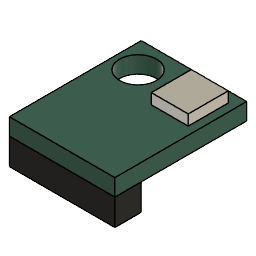
GREENHOUSE NEW VERSION (Autodesk Fusion 360 archive; units mm, degrees)
design "BMP180"
Autodesk Fusion 360 part; units mm, degrees
(part 1 of 25)
sketch "Sketch1" plane through (0, 0, 0) normal (0, 0, 1) x (1, 0, 0)
  line L0 (0, 0) -> (10, 0)
  line L1 (10, 0) -> (10, 12.5)
  line L2 (10, 12.5) -> (0, 12.5)
  line L3 (0, 12.5) -> (0, 0)
  circle A0 centre (2.25, 9.95) radius 1.75
  line L4 (5.75, 11.5) -> (9.25, 11.5)
  line L5 (9.25, 11.5) -> (9.25, 7.7)
  line L6 (9.25, 7.7) -> (5.75, 7.7)
  line L7 (5.75, 7.7) -> (5.75, 11.5)
  line L8 (10, 2.5) -> (0, 2.5)
  dimension "d1" = 10
  dimension "d2" = 12.5
  dimension "d3" = 3.5
  dimension "d4" = 2.55
  dimension "d5" = 2.25
  dimension "d6" = 3.5
  dimension "d7" = 3.8
  dimension "d8" = 0.75
  dimension "d9" = 1
  dimension "d10" = 2.5
  constraint horizontal L0
  constraint vertical L1
  constraint horizontal L2
  constraint vertical L3
  constraint coincident L0.start L3.end
  constraint horizontal L4
  constraint vertical L5
  constraint horizontal L6
  constraint vertical L7
  constraint coincident L1 L8.start
  constraint coincident L3 L8.end
  constraint perpendicular L3 L8
  measures "d1" distance of L0.start L0.end
  measures "d2" distance of L0.start L2.end
  measures "d3" diameter of A0
  measures "d4" distance of L2 A0.centre
  measures "d5" distance of L3 A0.centre
  measures "d6" distance of L4.start L4.end
  measures "d7" distance of L4.start L6.end
  measures "d8" distance of L1 L5
  measures "d9" distance of L2 L4
  measures "d10" distance of L0 L8
extrude "Extrude1" add sketch "Sketch1" along normal blind 1.6 contours L0 L1 L3 L8 | L1 L2 L3 L8 | L4 L5 L6 L7 makes body 1
extrude "Extrude2" add sketch "Sketch1" along normal blind 1 from surface at 1.6 separate body contours L4 L5 L6 L7 makes body 2
extrude "Extrude3" add sketch "Sketch1" against normal blind 2.5 separate body contours L0 L1 L3 L8 makes body 3
equation "d4 = d3 / 2 + 0.8 mm"
equation "d5 = d3 / 2 + 0.5 mm"

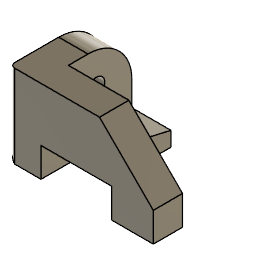
design "MOUNT REAl"
part number: 2026-05-05-22-33-46-720
Autodesk Fusion 360 part; units mm, degrees
sketch "Sketch1" plane through (0, 0, 0) normal (0, 0, 1) x (1, 0, 0)
  line L0 (0, 0) -> (14.68, 0)
  line L1 (14.68, 0) -> (14.68, 3)
  line L2 (14.68, 3) -> (11.68, 3)
  line L3 (11.68, 3) -> (3, 3)
  line L4 (3, 3) -> (3, 9.502)
  line L5 (0, 0) -> (0, 9.502)
  line L6 (0, 9.502) -> (3, 9.502)
  dimension "d4" = 3
  dimension "d5" = 3
  dimension "d6" = 8.68
  dimension "d7" = 6.502
  dimension "d88" = 3
  constraint coincident L0.start L5.start
  constraint horizontal L0
  constraint perpendicular L0 L1
  constraint perpendicular L1 L2
  constraint parallel L2 L3
  constraint perpendicular L3 L4
  constraint perpendicular L0 L5
  constraint perpendicular L4 L6
  measures "d4" distance of L0.end L1.end
  measures "d5" distance of L1.end L2.end
  measures "d6" distance of L2.end L3.end
  measures "d7" distance of L3.end L4.end
  measures "d88" distance of L4.end L5.end
extrude "Extrude18" add sketch "Sketch1" along normal blind 8.5 makes body 1
sketch "Sketch18" plane through (0, 0, 0) normal (0, -1, 0) x (1, 0, 0)
  line L0 (0, 0) -> (14.68, 0)
  line L1 (14.68, 0) -> (14.68, 8.5)
  line L2 (14.68, 8.5) -> (0, 8.5)
  line L3 (0, 8.5) -> (0, 0)
  line L4 (3.2, 0) -> (10.41, 0)
  line L5 (10.41, 0) -> (10.41, 3)
  line L6 (10.41, 3) -> (3.2, 3)
  line L7 (3.2, 3) -> (3.2, 0)
  dimension "d93" = 7.21
  dimension "d94" = 3
  dimension "d95" = 10.41
  constraint perpendicular L4 L5
  constraint perpendicular L5 L6
  constraint perpendicular L4 L7
  constraint coincident L0 L4.start
  constraint coincident L0 L4.end
  measures "d93" distance of L5.end L6.end
  measures "d94" distance of L4.end L5.end
  measures "d95" distance of L3 L5
extrude "Extrude19" cut sketch "Sketch18" against normal blind 3 contours L0 L4 L5 L6 L7 bodies 1
sketch "Sketch19" plane through (0, 0, 0) normal (0, 0, 1) x (1, 0, 0)
  line L0 (1.73, 2) -> (1.73, 8.5)
  line L1 (1.73, 8.5) -> (7.43, 8.5)
  line L2 (7.43, 8.5) -> (7.43, 2)
  line L3 (7.43, 2) -> (1.73, 2)
  dimension "d99" = 5.7
  constraint perpendicular L0 L1
  constraint perpendicular L1 L2
  measures "d99" distance of L0.end L1.end
sketch "Sketch23" plane through (0, 0, 0) normal (-1, 0, 0) x (0, -1, 0)
  line L0 (-9.502, 0) -> (0, 0)
  line L1 (0, 0) -> (0, 8.5)
  line L2 (0, 8.5) -> (-9.502, 8.5)
  line L3 (-9.502, 8.5) -> (-9.502, 0)
  circle A0 centre (-5.852, 5.15) radius 0.8695
  dimension "d107" = 1.739
  dimension "d108" = 3.35
  dimension "d109" = 3.65
  measures "d107" diameter of A0
  measures "d108" distance of L2 A0.centre
  measures "d109" distance of L3 A0.centre
extrude "Extrude23" cut sketch "Sketch23" against normal blind 6.5 contours A0 bodies 1
fillet "Fillet3" radius 4.5 1 edges at (1.5, 9.502, 8.5) on bodies 1
chamfer "Chamfer3" distance 0.5 angle 45 1 edges at (0, 4.751, 0) on bodies 1
fillet "Fillet4" radius 0.5 1 edges at (0, 0, 4.5) on bodies 1
chamfer "Chamfer4" distance 5.5 angle 45 1 edges at (14.68, 1.5, 8.5) on bodies 1
sketch "Sketch24" plane through (0, 0, 0) normal (0, 0, 1) x (1, 0, 0)
  line L0 (3, 3) -> (7, 3)
  line L1 (7, 3) -> (7, 9.5)
  line L2 (7, 9.5) -> (3, 9.5)
  line L3 (3, 9.5) -> (3, 3)
  dimension "d118" = 4
  dimension "d119" = 6.5
  dimension "d120" = 3
  dimension "d121" = 3
  constraint horizontal L0
  constraint perpendicular L0 L1
  constraint perpendicular L1 L2
  constraint perpendicular L0 L3
  measures "d118" distance of L0.start L0.end
  measures "d119" distance of L0 L2
  measures "d120" distance of origin L3
  measures "d121" distance of origin L0
extrude "Extrude24" add sketch "Sketch24" along normal blind 3 separate body makes body 2
sketch "Sketch25" plane through (7, 0, 0) normal (1, 0, 0) x (0, 1, 0)
  line L0 (3, 0) -> (9.5, 0)
  line L1 (9.5, 0) -> (9.5, 3)
  line L2 (9.5, 3) -> (3, 3)
  line L3 (3, 3) -> (3, 0)
  line L4 (3, 3) -> (9.5, 1.5)
  line L5 (9.5, 1.5) -> (3, 1.5)
  line L6 (3, 3) -> (3, 1.5)
  constraint coincident L2.end L3.start
  constraint midpoint L1 L4.end
  constraint midpoint L3 L5.end
extrude "Extrude25" cut sketch "Sketch25" against normal blind 2 contours L1 L2 L4 bodies 2
extrude "Extrude26" cut sketch "Sketch25" against normal blind 4 contours L1 L2 L4 bodies 2

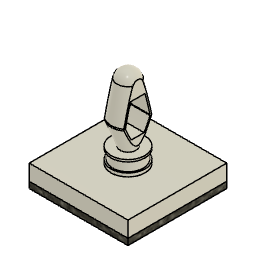
design "PCB Support Pin"
Autodesk Fusion 360 part; units mm, degrees
sketch "Sketch1" plane through (0, 0, 0) normal (0, 0, 1) x (1, 0, 0)
  line L0 (6.35, 6.35) -> (-6.35, 6.35)
  line L1 (-6.35, 6.35) -> (-6.35, -6.35)
  line L2 (-6.35, -6.35) -> (6.35, -6.35)
  line L3 (6.35, -6.35) -> (6.35, 6.35)
  line L4 (6.35, 6.35) -> (-6.35, -6.35) construction
  line L5 (-6.35, 6.35) -> (6.35, -6.35) construction
  dimension "d1" = 12.7
  dimension "d2" = 12.7
  constraint horizontal L0
  constraint perpendicular L0 L1
  constraint parallel L0 L2
  constraint parallel L1 L3
  constraint coincident L4 origin
  constraint coincident L5 origin
  measures "d1" distance of L1.end L2.end
  measures "d2" distance of L0.end L1.end
extrude "Extrude1" add sketch "Sketch1" along normal blind 2.032 makes body 1
extrude "Extrude2" add 1 faces at (-2.1167, -2.1167, 0) along direction (0, 0, -1) blind 0.8 separate body on bodies 1 makes body 2
sketch "Sketch2" plane through (0, 0, 0) normal (0, 1, 0) x (1, 0, 0)
  line L0 (-6.35, -2.032) -> (6.35, -2.032)
  line L1 (0, -2.032) -> (0, -12.6938)
  line L2 (0, -3.9625) -> (2.1828, -3.9625)
  line L3 (2.1828, -3.9625) -> (2.1828, -3.6971)
  line L4 (2.1828, -3.6971) -> (1.9857, -3.6971)
  line L5 (1.9857, -3.6971) -> (1.9857, -2.4654)
  line L6 (1.9857, -2.4654) -> (2.1828, -2.4654)
  line L7 (2.1828, -2.4654) -> (2.1828, -2.032)
  line L8 (6.35, 0.8) -> (-6.35, 0.8) construction
  line L9 (1.0176, -3.9625) -> (2.1587, -7.0975)
  line L10 (2.1763, -7.3064) -> (1.4028, -11.5248)
  arc A0 (0, -12.6938) -> (1.4028, -11.5248) centre (0, -11.2676) ccw
  arc A1 (2.1763, -7.3064) -> (2.1587, -7.0975) centre (1.7828, -7.2343) ccw
  line L11 (0, -12.6938) -> (1.1885, -12.6938) construction
  line L12 (1.1885, -12.6938) -> (1.4028, -11.5248) construction
  line L13 (2.1828, -3.9625) -> (2.1828, -7.2343) construction
  line L14 (1.6, -3.9625) -> (1.6, -5.5625) construction
  line L15 (1.6, -5.5625) -> (0, -5.5625) construction
  arc A2 (1.9795, -7.2704) -> (1.9708, -7.1659) centre (1.7828, -7.2343) ccw
  line L16 (0.8297, -4.0309) -> (0.8048, -3.9625)
  dimension "d7" = 4.7625
  dimension "d8" = 4.3656
  dimension "d10" = 0.4
  dimension "d11" = 8.7313
  dimension "d12" = 3.2
  dimension "d13" = 1.6
  dimension "d15" = 70
  constraint midpoint L0 L1.start
  constraint perpendicular L0 L1
  constraint perpendicular L1 L2
  constraint perpendicular L2 L3
  constraint perpendicular L3 L4
  constraint perpendicular L4 L5
  constraint perpendicular L5 L6
  constraint coincident L0 L7.end
  constraint perpendicular L0 L7
  constraint collinear L3 L7
  constraint coincident L2.start L1
  constraint coincident L1.end A0.start
  constraint tangent L10 A0
  constraint tangent L9 A1
  constraint tangent L10 A1
  constraint perpendicular L1 L11
  constraint tangent A0 L12
  constraint tangent A0 L11
  constraint coincident A1 L13.end
  constraint tangent A1 L13
  constraint perpendicular L2 L13
  constraint coincident L2 L9.start
  constraint coincident L2 L14.start
  constraint coincident L9 L14.end
  constraint perpendicular L2 L14
  constraint coincident L1 L15.end
  constraint perpendicular L1 L15
  constraint coincident L2 L16.end
  constraint concentric A1 A2
  measures "d7" distance of L2 L8
  measures "d10" radius of A1
  measures "d11" distance of L2 L1.end
  measures "d13" distance of L14.start L14.end
  measures "d15" angle of L2 L9
revolve "Revolve1" add sketch "Sketch2" angle 360 about axis through (0, 0, 2.032) along (0, 0, 1) bodies 1
sketch "Sketch3" plane through (0, 0, 0) normal (0, 1, 0) x (1, 0, 0)
  line L0 (-2.1828, -3.9625) -> (2.1828, -3.9625)
  arc A0 (-1.4028, -11.5248) -> (0, -12.6938) centre (0, -11.2676) ccw
  arc A1 (0, -12.6938) -> (1.4028, -11.5248) centre (0, -11.2676) ccw
  line L1 (1.25, -3.9625) -> (1.25, -12.6938)
  line L2 (1.25, -12.6938) -> (-1.25, -12.6938)
  line L3 (-1.25, -12.6938) -> (-1.25, -3.9625)
  line L4 (2.1828, -3.9625) -> (2.1828, -12.6938)
  line L5 (2.1828, -12.6938) -> (1.25, -12.6938)
  line L6 (-1.25, -12.6938) -> (-2.1828, -12.6938)
  line L7 (-2.1828, -12.6938) -> (-2.1828, -3.9625)
  dimension "d16" = 2.5
  constraint coincident L0 L1.start
  constraint perpendicular L0 L1
  constraint perpendicular L1 L2
  constraint coincident L0 L3.end
  constraint perpendicular L0 L3
  constraint midpoint A0.end L2
  constraint coincident L0.end L4.start
  constraint perpendicular L0 L4
  constraint perpendicular L1 L5
  constraint perpendicular L3 L6
  constraint coincident L0.start L7.end
  constraint perpendicular L0 L7
  measures "d16" distance of L1.end L2.end
extrude "Extrude3" cut sketch "Sketch3" along normal through all and the other way through all contours L0 L3 L6 L7 | L0 L1 L4 L5 bodies 1
sketch "Sketch4" plane through (1.25, 0, 0) normal (1, 0, 0) x (0, 1, 0)
  arc A0 (0.6367, 11.5248) -> (-0.6367, 11.5248) centre (0, 11.2676) ccw
  spline S0 degree 2 poles (-1.7815, 7.3064) (-1.0854, 10.4141) (-0.6367, 11.5248) knots 0 0 0 0.437351 0.437351 0.437351 weights 1 1.055449 1
  spline S1 degree 3 poles (-1.76, 7.0975) (-1.7782, 7.1383) (-1.7895, 7.19) (-1.7895, 7.2343) (-1.7895, 7.2572) (-1.7869, 7.2821) (-1.7815, 7.3064) knots -0.013287 -0.013287 -0.013287 -0.013287 0 0 0 0.006866 0.006866 0.006866 0.006866
  spline S2 degree 2 poles (0, 4.6009) (-0.6454, 4.6009) (-1.76, 7.0975) knots 0.311685 0.311685 0.311685 0.623369 0.623369 0.623369 weights 1 1.16768 1
  spline S3 degree 2 poles (1.76, 7.0975) (0.6454, 4.6009) (0, 4.6009) knots 0 0 0 0.311685 0.311685 0.311685 weights 1 1.16768 1
  spline S4 degree 3 poles (1.7815, 7.3064) (1.7869, 7.2821) (1.7895, 7.2572) (1.7895, 7.2343) (1.7895, 7.19) (1.7782, 7.1383) (1.76, 7.0975) knots -0.006866 -0.006866 -0.006866 -0.006866 0 0 0 0.013287 0.013287 0.013287 0.013287
  spline S5 degree 2 poles (0.6367, 11.5248) (1.0854, 10.4141) (1.7815, 7.3064) knots 0 0 0 0.437351 0.437351 0.437351 weights 1 1.055449 1
  spline S6 degree 3 poles (1.5773, 7.179) (1.0909, 6.0894) (0.7682, 5.5108) (0.4944, 5.1632) (0.2828, 4.8944) (0.1228, 4.8009) (0, 4.8009) knots 0 0 0 0 0.17577 0.17577 0.17577 0.311685 0.311685 0.311685 0.311685
  spline S7 degree 3 poles (0, 4.8009) (-0.1696, 4.8009) (-0.4174, 4.9925) (-0.7546, 5.5437) (-0.9772, 5.9076) (-1.2343, 6.4106) (-1.5773, 7.179) knots 0.311685 0.311685 0.311685 0.311685 0.499423 0.499423 0.499423 0.623369 0.623369 0.623369 0.623369
  spline S8 degree 3 poles (-1.5773, 7.179) (-1.5825, 7.1906) (-1.5895, 7.2239) (-1.5895, 7.2343) (-1.5895, 7.2423) (-1.5883, 7.2538) (-1.5863, 7.2627) knots -0.013287 -0.013287 -0.013287 -0.013287 0 0 0 0.006866 0.006866 0.006866 0.006866
  spline S9 degree 3 poles (-1.5863, 7.2627) (-1.1749, 9.0993) (-0.8714, 10.2577) (-0.6005, 11.0468) (-0.5494, 11.1956) (-0.4997, 11.3299) (-0.4512, 11.4499) knots 0 0 0 0 0.367958 0.367958 0.367958 0.437351 0.437351 0.437351 0.437351
  arc A1 (0.4512, 11.4499) -> (-0.4512, 11.4499) centre (0, 11.2676) ccw
  spline S10 degree 3 poles (0.4512, 11.4499) (0.7082, 10.8137) (0.9931, 9.8115) (1.3651, 8.2283) (1.4352, 7.9297) (1.5087, 7.6091) (1.5863, 7.2627) knots 0 0 0 0 0.367958 0.367958 0.367958 0.437351 0.437351 0.437351 0.437351
  spline S11 degree 3 poles (1.5863, 7.2627) (1.5883, 7.2538) (1.5895, 7.2423) (1.5895, 7.2343) (1.5895, 7.2239) (1.5825, 7.1906) (1.5773, 7.179) knots -0.006866 -0.006866 -0.006866 -0.006866 0 0 0 0.013287 0.013287 0.013287 0.013287
  line L0 (0.8161, 5.6442) -> (-0.8149, 5.6442)
  line L1 (0.9353, 9.9416) -> (-0.9355, 9.9416)
  dimension "d18" = 0.2
  constraint coincident S6 L0.start
  constraint coincident S7 L0.end
  constraint horizontal L0
  constraint coincident S10 L1.start
  constraint coincident S9 L1.end
  constraint parallel L0 L1
extrude "Extrude4" cut sketch "Sketch4" against normal through all contours S6 S7 S8 S9 S10 S11 L0 L1 bodies 1
equation "d7 = 3\" / 16"
equation "d8 = 11\" / 64"
equation "d11 = 11\" / 32"

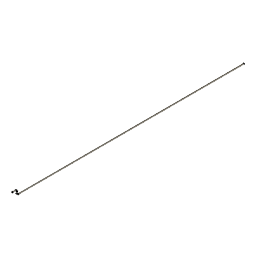
design "Push Rod"
Autodesk Fusion 360 part; units mm, degrees
sketch "Sketch1" plane through (0, 0, 0) normal (1, 0, 0) x (0, 1, 0)
  line L0 (0, 0) -> (3, 0)
  line L1 (4, -1) -> (4, -3)
  line L2 (5, -4) -> (204, -4)
  arc A0 (4, -1) -> (3, 0) centre (3, -1) ccw
  arc A1 (4, -3) -> (5, -4) centre (5, -3) ccw
  point P0 (4, 0)
  point P1 (4, -4)
  dimension "d1" = 4
  dimension "d2" = 4
  dimension "d3" = 200
  dimension "d4" = 1
  dimension "d5" = 1
  constraint coincident L0.start origin
  constraint horizontal L0
  constraint perpendicular L0 L1
  constraint perpendicular L1 L2
  constraint coincident P0 L0
  constraint coincident P0 L1
  constraint tangent L0 A0
  constraint tangent L1 A0
  constraint coincident P1 L1
  constraint coincident P1 L2
  constraint tangent L1 A1
  constraint tangent L2 A1
  measures "d1" distance of L0.start P0
  measures "d2" distance of P0 P1
  measures "d3" distance of P1 L2.end
  measures "d4" radius of A0
  measures "d5" radius of A1
sketch "Sketch2" plane through (0, 0, 0) normal (0, 1, 0) x (1, 0, 0)
  circle A0 centre (0, 0) radius 0.6
  dimension "d6" = 1.2
  constraint coincident A0.centre origin
  measures "d6" diameter of A0
sweep "Sweep1" add profiles "Sketch2" path "Sketch1" along L0 A0 L1 A1 L2 section 1

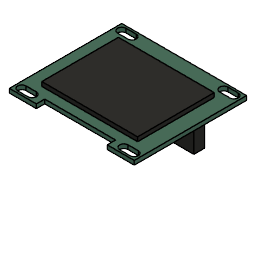
design "oled"
description: IIC OLED 0.96" 4Pin SSD1306
part number: GME12864-11
Autodesk Fusion 360 part; units mm, degrees
sketch "Sketch1" plane through (0, 0, 0) normal (0, 1, 0) x (1, 0, 0)
  line L0 (0, 0) -> (30, 0)
  line L1 (30, 0) -> (30, -27)
  line L2 (30, -27) -> (0, -27)
  line L3 (0, -27) -> (0, 0)
  line L4 (6.5, -27) -> (6.5, -25)
  line L5 (6.5, -25) -> (23.5, -25)
  line L6 (23.5, -25) -> (23.5, -27)
  line L7 (15, -27) -> (15, -25) construction
  line L8 (3.5, -4.3) -> (26.5, -4.3)
  line L9 (26.5, -4.3) -> (26.5, -22.7)
  line L10 (26.5, -22.7) -> (3.5, -22.7)
  line L11 (3.5, -22.7) -> (3.5, -4.3)
  line L12 (1.5, -2.5) -> (4, -2.5)
  arc A0 (4, -2.5) -> (4, -0.5) centre (4, -1.5) ccw
  line L13 (4, -0.5) -> (1.5, -0.5)
  arc A1 (1.5, -0.5) -> (1.5, -2.5) centre (1.5, -1.5) ccw
  line L14 (1.5, -1.5) -> (4, -1.5) construction
  line L15 (15, 0) -> (15, -25) construction
  line L16 (0, -13.5) -> (30, -13.5) construction
  arc A2 (26, -0.5) -> (26, -2.5) centre (26, -1.5) ccw
  line L17 (26, -0.5) -> (28.5, -0.5)
  arc A3 (28.5, -2.5) -> (28.5, -0.5) centre (28.5, -1.5) ccw
  line L18 (28.5, -2.5) -> (26, -2.5)
  line L19 (26, -26.5) -> (28.5, -26.5)
  arc A4 (28.5, -26.5) -> (28.5, -24.5) centre (28.5, -25.5) ccw
  line L20 (28.5, -24.5) -> (26, -24.5)
  arc A5 (26, -24.5) -> (26, -26.5) centre (26, -25.5) ccw
  line L21 (4, -26.5) -> (1.5, -26.5)
  arc A6 (4, -26.5) -> (4, -24.5) centre (4, -25.5) ccw
  arc A7 (1.5, -24.5) -> (1.5, -26.5) centre (1.5, -25.5) ccw
  line L22 (1.5, -24.5) -> (4, -24.5)
  dimension "d1" = 30
  dimension "d2" = 27
  dimension "d3" = 6.5
  dimension "d4" = 2
  dimension "d5" = 3.5
  dimension "d6" = 3.5
  dimension "d7" = 4.3
  dimension "d8" = 4.3
  dimension "d22" = 1.5
  dimension "d23" = 1.5
  dimension "d24" = 1
  dimension "d25" = 2.5
  constraint horizontal L0
  constraint vertical L1
  constraint horizontal L2
  constraint vertical L3
  constraint coincident L0.start L3.end
  constraint coincident L2 L4.start
  constraint perpendicular L2 L4
  constraint perpendicular L4 L5
  constraint coincident L2 L6.end
  constraint perpendicular L2 L6
  constraint midpoint L2 L7.start
  constraint midpoint L5 L7.end
  constraint perpendicular L2 L7
  constraint horizontal L8
  constraint vertical L9
  constraint horizontal L10
  constraint vertical L11
  constraint tangent L12 A0
  constraint tangent A0 L13
  constraint parallel L12 L13
  constraint tangent L13 A1
  constraint tangent L12 A1
  constraint horizontal L14
  constraint midpoint L0 L15.start
  constraint midpoint L3 L16.start
  constraint midpoint L1 L16.end
  constraint symmetric L12.start L15 A3.start
  constraint symmetric L12.end L15 A2.end
  constraint symmetric A0.end L15 A2.start
  constraint symmetric L13.end L15 L17.end
  constraint symmetric A0 L15 A2
  constraint symmetric A1 L15 A3
  constraint symmetric L12.start L16 A7.start
  constraint symmetric L12.end L16 A6.end
  constraint symmetric A0.end L16 L21.start
  constraint symmetric L13.end L16 L21.end
  constraint symmetric A0 L16 A6
  constraint symmetric A1 L16 A7
  constraint symmetric L16 A2.end L20.end
  constraint symmetric L16 A2.start L19.start
  constraint symmetric L16 A2 A5
  constraint symmetric L16 L17.end L19.end
  constraint symmetric L16 A3.start A4.end
  constraint symmetric L16 A3 A4
  measures "d1" distance of L0.start L0.end
  measures "d2" distance of L0.start L2.end
  measures "d3" distance of L1 L6
  measures "d4" distance of L2 L5
  measures "d5" distance of L1 L9
  measures "d6" distance of L3 L11
  measures "d7" distance of L0 L8
  measures "d8" distance of L2 L10
  measures "d22" distance of L3 A1.centre
  measures "d23" distance of L0 A1.centre
  measures "d24" radius of A1
  measures "d25" distance of A1.centre A0.centre
extrude "Extrude1" add sketch "Sketch1" along normal blind 1 contours L8 L9 L10 L11 makes body 1
extrude "Extrude2" add sketch "Sketch1" against normal blind 1 separate body contours L0 L1 L2 L3 L4 L5 L6 | L8 L9 L10 L11 makes body 2
sketch "Sketch2" plane through (0, -1, 0) normal (0, -1, 0) x (1, 0, 0)
  line L0 (6.5, 25) -> (6.5, 27)
  line L1 (6.5, 27) -> (0, 27)
  line L2 (0, 27) -> (0, 0)
  line L3 (0, 0) -> (30, 0)
  line L4 (30, 0) -> (30, 27)
  line L5 (30, 27) -> (23.5, 27)
  line L6 (23.5, 27) -> (23.5, 25)
  line L7 (23.5, 25) -> (6.5, 25)
  line L8 (10.1, 2.6) -> (19.9, 2.6)
  line L9 (19.9, 2.6) -> (19.9, 0)
  line L10 (10.1, 0) -> (10.1, 2.6)
  line L11 (15, 0) -> (15, 2.6) construction
  arc A0 (26, 2.5) -> (26, 0.5) centre (26, 1.5) ccw
  line L12 (26, 2.5) -> (28.5, 2.5)
  arc A1 (28.5, 0.5) -> (28.5, 2.5) centre (28.5, 1.5) ccw
  line L13 (28.5, 0.5) -> (26, 0.5)
  arc A2 (26, 26.5) -> (26, 24.5) centre (26, 25.5) ccw
  line L14 (26, 26.5) -> (28.5, 26.5)
  arc A3 (28.5, 24.5) -> (28.5, 26.5) centre (28.5, 25.5) ccw
  line L15 (28.5, 24.5) -> (26, 24.5)
  arc A4 (4, 24.5) -> (4, 26.5) centre (4, 25.5) ccw
  line L16 (4, 24.5) -> (1.5, 24.5)
  arc A5 (1.5, 26.5) -> (1.5, 24.5) centre (1.5, 25.5) ccw
  line L17 (1.5, 26.5) -> (4, 26.5)
  arc A6 (1.5, 2.5) -> (1.5, 0.5) centre (1.5, 1.5) ccw
  line L18 (1.5, 2.5) -> (4, 2.5)
  arc A7 (4, 0.5) -> (4, 2.5) centre (4, 1.5) ccw
  line L19 (4, 0.5) -> (1.5, 0.5)
  dimension "d13" = 9.8
  dimension "d14" = 2.6
  constraint horizontal L8
  constraint vertical L9
  constraint vertical L10
  constraint midpoint L3 L11.start
  constraint perpendicular L3 L11
  constraint coincident L3 L9.end
  constraint coincident L3 L10.start
  constraint midpoint L8 L11.end
  measures "d13" distance of L8.start L8.end
  measures "d14" distance of L8.start L10.start
extrude "Extrude3" add sketch "Sketch2" along normal blind 15 separate body contours L3 L8 L9 L10 makes body 3
sketch "Minimal Projection" plane through (0, -1, 0) normal (0, -1, 0) x (1, 0, 0)
  arc A0 (26, 2.5) -> (26, 0.5) centre (26, 1.5) ccw
  line L0 (26, 2.5) -> (28.5, 2.5)
  arc A1 (28.5, 0.5) -> (28.5, 2.5) centre (28.5, 1.5) ccw
  line L1 (28.5, 0.5) -> (26, 0.5)
  arc A2 (26, 26.5) -> (26, 24.5) centre (26, 25.5) ccw
  line L2 (26, 26.5) -> (28.5, 26.5)
  arc A3 (28.5, 24.5) -> (28.5, 26.5) centre (28.5, 25.5) ccw
  line L3 (28.5, 24.5) -> (26, 24.5)
  arc A4 (4, 24.5) -> (4, 26.5) centre (4, 25.5) ccw
  line L4 (4, 24.5) -> (1.5, 24.5)
  arc A5 (1.5, 26.5) -> (1.5, 24.5) centre (1.5, 25.5) ccw
  line L5 (1.5, 26.5) -> (4, 26.5)
  arc A6 (1.5, 2.5) -> (1.5, 0.5) centre (1.5, 1.5) ccw
  line L6 (1.5, 2.5) -> (4, 2.5)
  arc A7 (4, 0.5) -> (4, 2.5) centre (4, 1.5) ccw
  line L7 (4, 0.5) -> (1.5, 0.5)
  line L8 (6.5, 25) -> (6.5, 27)
  line L9 (6.5, 27) -> (0, 27)
  line L10 (0, 27) -> (0, 0)
  line L11 (0, 0) -> (30, 0)
  line L12 (30, 0) -> (30, 27)
  line L13 (30, 27) -> (23.5, 27)
  line L14 (23.5, 27) -> (23.5, 25)
  line L15 (23.5, 25) -> (6.5, 25)
  line L16 (19.9, 0) -> (19.9, 2.6)
  line L17 (19.9, 2.6) -> (10.1, 2.6)
  line L18 (10.1, 2.6) -> (10.1, 0)

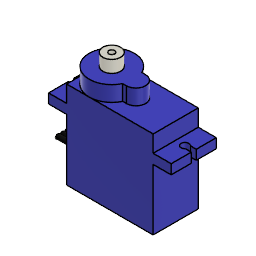
design "SG90 Micro Servo"
Autodesk Fusion 360 part; units mm, degrees
sketch "Sketch2" plane through (0, 0, 0) normal (0, 1, 0) x (1, 0, 0)
  line L0 (0, 0) -> (22.5, 0)
  line L1 (22.5, 0) -> (22.5, -22.75)
  line L2 (22.5, -22.75) -> (0, -22.75)
  line L3 (0, -22.75) -> (0, 0)
  line L4 (-4.7, -15.9) -> (-4.7, -18.4)
  line L5 (27.2, -18.4) -> (27.2, -15.9)
  line L6 (-4.7, -18.4) -> (0, -18.4)
  line L7 (22.5, -18.4) -> (27.2, -18.4)
  line L8 (27.2, -15.9) -> (22.5, -15.9)
  line L9 (0, -15.9) -> (-4.7, -15.9)
  dimension "d3" = 22.5
  dimension "d4" = 22.75
  dimension "d6" = 4.35
  dimension "d7" = 2.5
  dimension "d8" = 4.7
  dimension "d9" = 4.7
  constraint horizontal L0
  constraint vertical L1
  constraint horizontal L2
  constraint vertical L3
  constraint coincident L0.start L3.end
  constraint horizontal L8
  constraint vertical L4
  constraint horizontal L6
  constraint vertical L5
  constraint coincident L3 L6.end
  constraint coincident L1 L7.start
  constraint collinear L6 L7
  constraint coincident L1 L8.end
  constraint coincident L3 L9.start
  constraint collinear L8 L9
  measures "d3" distance of L0.start L0.end
  measures "d4" distance of L0.start L2.end
  measures "d6" distance of L2 L6
  measures "d7" distance of L5.end L5.start
  measures "d8" distance of L1 L5
  measures "d9" distance of L3 L4
extrude "Extrude2" add sketch "Sketch2" along normal blind 11.75 makes body 1
sketch "Sketch3" plane through (0, 0, 22.75) normal (0, 0, 1) x (-1, 0, 0)
  line L0 (0, 0) -> (-22.5, 0)
  line L1 (-22.5, 0) -> (-22.5, -11.75)
  line L2 (-22.5, -11.75) -> (0, -11.75)
  line L3 (0, -11.75) -> (0, 0)
  circle A0 centre (-5.875, -5.875) radius 5.875
  line L4 (-5.875, -5.875) -> (-12.175, -5.875) construction
  line L5 (-11.1915, -8.375) -> (-12.175, -8.375)
  line L6 (-11.1915, -3.375) -> (-12.175, -3.375)
  arc A1 (-12.175, -3.375) -> (-12.175, -8.375) centre (-12.175, -5.875) ccw
  dimension "d13" = 6.3
  dimension "d14" = 2.5
  constraint tangent L0 A0
  constraint tangent L2 A0
  constraint tangent L3 A0
  constraint coincident A0.centre L4.start
  constraint coincident L4.end A1.centre
  constraint horizontal L4
  constraint coincident A0 L5.start
  constraint tangent L5 A1
  constraint coincident A0 L6.start
  constraint tangent L6 A1
  constraint horizontal L5
  constraint horizontal L6
  measures "d13" distance of A0.centre L4.end
  measures "d14" radius of A1
extrude "Extrude3" add sketch "Sketch3" along normal blind 4 contours A0 | A0 L5 L6 A1 bodies 1
sketch "Sketch4" plane through (0, 0, 26.75) normal (0, 0, 1) x (-1, 0, 0)
  arc A0 (-11.1915, -8.375) -> (-11.1915, -3.375) centre (-5.875, -5.875) ccw
  line L0 (-11.1915, -3.375) -> (-12.175, -3.375)
  arc A1 (-12.175, -3.375) -> (-12.175, -8.375) centre (-12.175, -5.875) ccw
  line L1 (-12.175, -8.375) -> (-11.1915, -8.375)
  circle A2 centre (-5.875, -5.875) radius 2.3
  circle A3 centre (-5.875, -5.875) radius 0.75
  dimension "d17" = 4.6
  dimension "d28" = 1.5
  constraint concentric A0 A2
  constraint concentric A2 A3
  measures "d17" diameter of A2
  measures "d28" diameter of A3
extrude "Extrude4" add sketch "Sketch4" along normal blind 3.15 separate body contours A2 makes body 2
sketch "Sketch5" plane through (0, 0, 18.4) normal (0, 0, 1) x (-1, 0, 0)
  line L0 (4.7, 0) -> (0, 0)
  line L1 (0, 0) -> (0, -11.75)
  line L2 (0, -11.75) -> (4.7, -11.75)
  line L3 (4.7, -11.75) -> (4.7, 0)
  line L4 (-22.5, 0) -> (-27.2, 0)
  line L5 (-27.2, 0) -> (-27.2, -11.75)
  line L6 (-27.2, -11.75) -> (-22.5, -11.75)
  line L7 (-22.5, -11.75) -> (-22.5, 0)
  line L8 (-27.2, -5.875) -> (4.7, -5.875) construction
  line L9 (-11.25, -5.875) -> (-11.25, -0.3179)
  line L10 (4.7, -6.525) -> (3.1599, -6.525)
  line L11 (4.7, -5.225) -> (3.1599, -5.225)
  arc A0 (3.1599, -5.225) -> (3.1599, -6.525) centre (2.4, -5.875) ccw
  arc A1 (-25.6599, -6.525) -> (-25.6599, -5.225) centre (-24.9, -5.875) ccw
  line L12 (-27.2, -5.225) -> (-25.6599, -5.225)
  line L13 (-27.2, -6.525) -> (-25.6599, -6.525)
  dimension "d20" = 2
  dimension "d21" = 1.3
  dimension "d22" = 2.3
  constraint midpoint L5 L8.start
  constraint midpoint L3 L8.end
  constraint midpoint L8 L9.start
  constraint perpendicular L8 L9
  constraint coincident L8 A0.centre
  constraint coincident L3 L10.start
  constraint perpendicular L3 L10
  constraint coincident L3 L11.start
  constraint perpendicular L3 L11
  constraint symmetric L8 L10 L11
  constraint symmetric L9 L10.start L13.start
  constraint symmetric L9 L10.end A1.start
  constraint symmetric L9 L11.start L12.start
  constraint symmetric L9 L11.end A1.end
  constraint symmetric L9 A0 A1
  measures "d20" diameter of A0
  measures "d21" distance of L10 L11
  measures "d22" distance of L3 A0.centre
extrude "Extrude5" cut sketch "Sketch5" against normal through all contours L3 L10 L11 A0 | L5 A1 L12 L13 bodies 1
sketch "Sketch6" plane through (0, 0, 0) normal (-1, 0, 0) x (0, -1, 0)
  line L0 (0, 0) -> (0, 15.9)
  line L1 (0, 15.9) -> (-11.75, 15.9)
  line L2 (-11.75, 15.9) -> (-11.75, 0)
  line L3 (-11.75, 0) -> (0, 0)
  line L4 (-4.075, 5.7) -> (-7.675, 5.7) construction
  line L5 (-7.675, 5.7) -> (-7.675, 4.5) construction
  line L6 (-7.675, 4.5) -> (-4.075, 4.5) construction
  line L7 (-4.075, 4.5) -> (-4.075, 5.7) construction
  line L8 (-5.875, 4.5) -> (-5.875, 0) construction
  circle A0 centre (-5.875, 5.1) radius 0.6
  circle A1 centre (-4.675, 5.1) radius 0.6
  circle A2 centre (-7.075, 5.1) radius 0.6
  dimension "d24" = 1.2
  dimension "d25" = 4.5
  constraint horizontal L4
  constraint vertical L5
  constraint horizontal L6
  constraint vertical L7
  constraint midpoint L6 L8.start
  constraint coincident L3 L8.end
  constraint perpendicular L3 L8
  constraint midpoint L3 L8.end
  constraint tangent L4 A0
  constraint coincident L8.start A0
  constraint tangent L4 A1
  constraint tangent L7 A1
  constraint tangent L6 A1
  constraint tangent L4 A2
  constraint tangent L5 A2
  constraint tangent L6 A2
  constraint tangent A0 A1
  constraint tangent A0 A2
  measures "d24" distance of L4.start L6.end
  measures "d25" distance of L8.start L8.end
extrude "Extrude6" add sketch "Sketch6" along normal blind 7 separate body contours A0 | A2 | A1 makes body 3
equation "d43 = 3.9 mm - 2.2 mm"
named bodies: "Body", "Wires", "Mount"

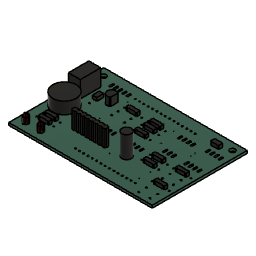
design "IO Daughter Board"
Autodesk Fusion 360 part; units mm, degrees
sketch "Outline" plane through (0, 0, 0) normal (0, 0, 1) x (1, 0, 0)
  line L0 (0, 0) -> (0, 56.3)
  arc A0 (0, 56.3381) -> (0, 56.2619) centre (0, 56.3) ccw
  line L1 (85, 56.3) -> (85, 0)
  arc A1 (85.0381, 56.3) -> (84.9619, 56.3) centre (85, 56.3) ccw
  arc A2 (0.0381, 56.3) -> (-0.0381, 56.3) centre (0, 56.3) ccw
  arc A3 (-0.0381, 0) -> (0.0381, 0) centre (0, 0) ccw
  line L2 (0, 56.3) -> (85, 56.3)
  arc A4 (0, 0.0381) -> (0, -0.0381) centre (0, 0) ccw
  arc A5 (85, 56.2619) -> (85, 56.3381) centre (85, 56.3) ccw
  arc A6 (85, -0.0381) -> (85, 0.0381) centre (85, 0) ccw
  line L3 (85, 0) -> (0, 0)
  arc A7 (84.9619, 0) -> (85.0381, 0) centre (85, 0) ccw
sketch "Top SIlkscreen" plane through (0, 0, 0) normal (0, 0, 1) x (1, 0, 0)
  line L0 (55.2958, 9.3303) -> (56.4642, 9.7197)
  arc A0 (55.2878, 9.3544) -> (55.3038, 9.3062) centre (55.2958, 9.3303) ccw
  arc A1 (52.7304, 13.311) -> (52.7812, 13.311) centre (52.7558, 13.311) ccw
  line L1 (56.1721, 9.6224) -> (56.1721, 9.0382)
  arc A2 (56.4722, 9.6956) -> (56.4562, 9.7438) centre (56.4642, 9.7197) ccw
  arc A3 (53.6646, 12.8425) -> (53.6646, 12.7917) centre (53.6646, 12.8171) ccw
  arc A4 (53.9242, 13.2856) -> (53.9242, 13.3364) centre (53.9242, 13.311) ccw
  arc A5 (53.9242, 10.5777) -> (53.9242, 10.6285) centre (53.9242, 10.6031) ccw
  arc A6 (53.6392, 10.1487) -> (53.69, 10.1487) centre (53.6646, 10.1487) ccw
  arc A7 (52.6347, 11.7855) -> (52.6173, 11.7377) centre (52.626, 11.7616) ccw
  arc A8 (53.8988, 12.5575) -> (53.9496, 12.5575) centre (53.9242, 12.5575) ccw
  arc A9 (52.7304, 12.4601) -> (52.7812, 12.4601) centre (52.7558, 12.4601) ccw
  line L2 (53.4049, 10.6031) -> (53.9242, 10.6031)
  arc A10 (53.7619, 12.168) -> (53.9242, 12.5575) centre (53.3757, 12.5575) ccw
  arc A11 (53.8988, 13.6356) -> (53.9496, 13.6356) centre (53.9242, 13.6356) ccw
  arc A12 (52.7638, 14.8408) -> (52.7478, 14.7926) centre (52.7558, 14.8167) ccw
  line L3 (53.9242, 13.6356) -> (53.9242, 13.311)
  arc A13 (52.8532, 12.7522) -> (52.7558, 12.4601) centre (53.2426, 12.4601) ccw
  arc A14 (53.0154, 12.1751) -> (53.0154, 12.2259) centre (53.0154, 12.2005) ccw
  arc A15 (53.6646, 12.8171) -> (53.4374, 12.6873) centre (53.6646, 12.5534) ccw
  line L4 (52.7558, 14.8167) -> (53.9242, 15.2061)
  arc A16 (53.9162, 14.4031) -> (53.9322, 14.4513) centre (53.9242, 14.4272) ccw
  arc A17 (53.69, 10.7978) -> (53.6392, 10.7978) centre (53.6646, 10.7978) ccw
  arc A18 (54.0453, 11.2184) -> (54.0627, 11.2662) centre (54.054, 11.2423) ccw
  arc A19 (53.0804, 13.9347) -> (53.0804, 13.9855) centre (53.0804, 13.9601) ccw
  arc A20 (53.8988, 13.311) -> (53.9496, 13.311) centre (53.9242, 13.311) ccw
  line L5 (56.4642, 8.9408) -> (55.2958, 9.3303)
  arc A21 (52.7812, 13.6356) -> (52.7304, 13.6356) centre (52.7558, 13.6356) ccw
  line L6 (53.9242, 14.4272) -> (52.7558, 14.8167)
  line L7 (53.6321, 15.1088) -> (53.6321, 14.5246)
  arc A22 (52.8735, 12.737) -> (52.8328, 12.7674) centre (52.8531, 12.7522) ccw
  arc A23 (53.0804, 13.9855) -> (53.0804, 13.9347) centre (53.0804, 13.9601) ccw
  arc A24 (55.3038, 9.3544) -> (55.2878, 9.3062) centre (55.2958, 9.3303) ccw
  arc A25 (53.744, 12.186) -> (53.7798, 12.15) centre (53.7619, 12.168) ccw
  arc A26 (53.0154, 12.2005) -> (53.2426, 12.3303) centre (53.0154, 12.4642) ccw
  arc A27 (52.7628, 10.4328) -> (52.7488, 10.3839) centre (52.7558, 10.4084) ccw
  arc A28 (52.7558, 12.4601) -> (53.0154, 12.2005) centre (53.0154, 12.4601) ccw
  line L8 (53.9242, 13.311) -> (52.7558, 13.311)
  arc A29 (53.2203, 12.3424) -> (53.2649, 12.3181) centre (53.2426, 12.3302) ccw
  arc A30 (52.7812, 12.4601) -> (52.7304, 12.4601) centre (52.7558, 12.4601) ccw
  arc A31 (53.4049, 10.6285) -> (53.4049, 10.5777) centre (53.4049, 10.6031) ccw
  arc A32 (53.0154, 12.2259) -> (53.0154, 12.1751) centre (53.0154, 12.2005) ccw
  arc A33 (52.7304, 13.6356) -> (52.7812, 13.6356) centre (52.7558, 13.6356) ccw
  line L9 (53.0804, 13.9601) -> (53.5996, 13.9601)
  arc A34 (53.9496, 12.5575) -> (53.8988, 12.5575) centre (53.9242, 12.5575) ccw
  arc A35 (53.5996, 13.9855) -> (53.5996, 13.9347) centre (53.5996, 13.9601) ccw
  arc A36 (53.5996, 13.9347) -> (53.5996, 13.9855) centre (53.5996, 13.9601) ccw
  line L10 (53.4374, 12.6873) -> (53.2426, 12.3303)
  arc A37 (53.0804, 13.9601) -> (52.7558, 13.6356) centre (53.0804, 13.6355) ccw
  arc A38 (53.9242, 13.6356) -> (53.5996, 13.9601) centre (53.5996, 13.6355) ccw
  arc A39 (53.9242, 12.5575) -> (53.6646, 12.8171) centre (53.6646, 12.5575) ccw
  arc A40 (53.2645, 12.3174) -> (53.2208, 12.3432) centre (53.2427, 12.3303) ccw
  arc A41 (53.4155, 12.7002) -> (53.4593, 12.6744) centre (53.4374, 12.6873) ccw
  arc A42 (53.4597, 12.6751) -> (53.4151, 12.6995) centre (53.4374, 12.6873) ccw
  arc A43 (53.9322, 15.182) -> (53.9162, 15.2302) centre (53.9242, 15.2061) ccw
  arc A44 (56.4562, 8.9167) -> (56.4722, 8.9649) centre (56.4642, 8.9408) ccw
  arc A45 (53.6646, 12.7917) -> (53.6646, 12.8425) centre (53.6646, 12.8171) ccw
  arc A46 (52.7478, 14.8408) -> (52.7638, 14.7926) centre (52.7558, 14.8167) ccw
  line L11 (54.054, 11.2423) -> (52.626, 11.7616)
  arc A47 (53.6575, 15.1088) -> (53.6067, 15.1088) centre (53.6321, 15.1088) ccw
  line L12 (52.7558, 13.311) -> (52.7558, 13.6356)
  arc A48 (52.7558, 13.3364) -> (52.7558, 13.2856) centre (52.7558, 13.311) ccw
  arc A49 (53.6067, 14.5246) -> (53.6575, 14.5246) centre (53.6321, 14.5246) ccw
  arc A50 (53.9496, 13.6356) -> (53.8988, 13.6356) centre (53.9242, 13.6356) ccw
  arc A51 (55.3212, 12.4601) -> (55.2704, 12.4601) centre (55.2958, 12.4601) ccw
  arc A52 (56.4642, 10.5382) -> (56.2046, 10.7978) centre (56.2046, 10.5382) ccw
  arc A53 (56.2046, 10.7724) -> (56.2046, 10.8232) centre (56.2046, 10.7978) ccw
  arc A54 (41.0619, 54.9233) -> (41.2242, 55.1504) centre (40.9841, 55.1504) ccw
  arc A55 (56.2046, 12.8425) -> (56.2046, 12.7917) centre (56.2046, 12.8171) ccw
  arc A56 (41.0537, 54.9473) -> (41.0702, 54.8992) centre (41.062, 54.9233) ccw
  line L13 (56.4642, 10.1487) -> (56.4642, 10.5382)
  arc A57 (56.4388, 12.5575) -> (56.4896, 12.5575) centre (56.4642, 12.5575) ccw
  arc A58 (41.1988, 55.1504) -> (41.2496, 55.1504) centre (41.2242, 55.1504) ccw
  arc A59 (55.2958, 10.1741) -> (55.2958, 10.1233) centre (55.2958, 10.1487) ccw
  arc A60 (40.64, 54.8513) -> (40.64, 54.8005) centre (40.64, 54.8259) ccw
  arc A61 (56.0747, 10.7724) -> (56.0747, 10.8232) centre (56.0747, 10.7978) ccw
  arc A62 (41.2242, 55.1504) -> (41.0619, 55.3776) centre (40.984, 55.1504) ccw
  arc A63 (41.0508, 55.3548) -> (41.0731, 55.4005) centre (41.0619, 55.3777) ccw
  arc A64 (55.7897, 10.1487) -> (55.8405, 10.1487) centre (55.8151, 10.1487) ccw
  arc A65 (55.3212, 10.7978) -> (55.2704, 10.7978) centre (55.2958, 10.7978) ccw
  arc A66 (56.4388, 10.1487) -> (56.4896, 10.1487) centre (56.4642, 10.1487) ccw
  line L14 (55.2958, 10.1487) -> (55.2958, 10.7978)
  arc A67 (56.4642, 12.5575) -> (56.2046, 12.8171) centre (56.2046, 12.5575) ccw
  arc A68 (34.8822, 28.7456) -> (34.8662, 28.7938) centre (34.8742, 28.7697) ccw
  arc A69 (40.64, 55.5004) -> (40.64, 55.4496) centre (40.64, 55.475) ccw
  arc A70 (56.4896, 10.5382) -> (56.4388, 10.5382) centre (56.4642, 10.5382) ccw
  arc A71 (56.3019, 12.168) -> (56.4642, 12.5575) centre (55.9157, 12.5575) ccw
  arc A72 (55.1747, 11.7855) -> (55.1573, 11.7377) centre (55.166, 11.7616) ccw
  arc A73 (55.5554, 12.1751) -> (55.5554, 12.2259) centre (55.5554, 12.2005) ccw
  arc A74 (56.2046, 10.8232) -> (56.2046, 10.7724) centre (56.2046, 10.7978) ccw
  arc A75 (55.8405, 10.5382) -> (55.7897, 10.5382) centre (55.8151, 10.5382) ccw
  arc A76 (41.0702, 55.4017) -> (41.0537, 55.3536) centre (41.0619, 55.3777) ccw
  arc A77 (55.8151, 10.1233) -> (55.8151, 10.1741) centre (55.8151, 10.1487) ccw
  line L15 (56.594, 11.2423) -> (55.166, 11.7616)
  line L16 (55.8151, 10.5382) -> (55.8151, 10.1487)
  arc A78 (40.9487, 54.871) -> (40.9804, 54.9106) centre (40.9646, 54.8908) ccw
  line L17 (40.9646, 54.8908) -> (40.3154, 55.4101)
  arc A79 (41.0619, 55.3776) -> (40.64, 55.475) centre (40.6399, 54.5123) ccw
  arc A80 (40.3313, 55.4299) -> (40.2996, 55.3903) centre (40.3154, 55.4101) ccw
  line L18 (43.7642, 52.5018) -> (42.5958, 52.5018)
  line L19 (42.5958, 52.5018) -> (42.5958, 52.8264)
  arc A81 (56.0747, 10.8232) -> (56.0747, 10.7724) centre (56.0747, 10.7978) ccw
  arc A82 (55.2704, 10.1487) -> (55.3212, 10.1487) centre (55.2958, 10.1487) ccw
  line L20 (56.2046, 10.7978) -> (56.0747, 10.7978)
  arc A83 (56.1975, 9.6224) -> (56.1467, 9.6224) centre (56.1721, 9.6224) ccw
  arc A84 (56.0747, 10.7978) -> (55.8151, 10.5382) centre (56.0747, 10.5382) ccw
  line L21 (55.8151, 10.1487) -> (55.2958, 10.1487)
  arc A85 (55.2958, 12.4601) -> (55.5554, 12.2005) centre (55.5554, 12.4601) ccw
  arc A86 (55.3932, 12.7522) -> (55.2958, 12.4601) centre (55.7826, 12.4601) ccw
  arc A87 (56.284, 12.186) -> (56.3198, 12.15) centre (56.3019, 12.168) ccw
  line L22 (26.6051, 29.6644) -> (26.6051, 29.2749)
  arc A88 (56.4896, 12.5575) -> (56.4388, 12.5575) centre (56.4642, 12.5575) ccw
  arc A89 (40.64, 55.4496) -> (40.64, 55.5004) centre (40.64, 55.475) ccw
  arc A90 (40.2069, 55.4005) -> (40.2292, 55.3548) centre (40.218, 55.3777) ccw
  arc A91 (41.0731, 54.9004) -> (41.0508, 54.9461) centre (41.062, 54.9233) ccw
  arc A92 (56.4388, 10.5382) -> (56.4896, 10.5382) centre (56.4642, 10.5382) ccw
  line L23 (43.9972, 30.4165) -> (44.6322, 30.4165)
  arc A93 (40.0304, 55.1504) -> (40.0812, 55.1504) centre (40.0558, 55.1504) ccw
  arc A94 (41.2496, 55.1504) -> (41.1988, 55.1504) centre (41.2242, 55.1504) ccw
  line L24 (29.1451, 28.4452) -> (29.1451, 28.6399)
  arc A95 (56.5853, 11.2184) -> (56.6027, 11.2662) centre (56.594, 11.2423) ccw
  arc A96 (47.9679, 10.7724) -> (47.9679, 10.8232) centre (47.9679, 10.7978) ccw
  line L25 (26.6051, 29.2749) -> (26.0858, 29.2749)
  arc A97 (40.64, 55.475) -> (40.2181, 55.3776) centre (40.6401, 54.5123) ccw
  arc A98 (56.1467, 9.0382) -> (56.1975, 9.0382) centre (56.1721, 9.0382) ccw
  arc A99 (40.64, 54.8259) -> (41.0619, 54.9233) centre (40.6399, 55.7886) ccw
  arc A100 (55.7897, 10.5382) -> (55.8405, 10.5382) centre (55.8151, 10.5382) ccw
  arc A101 (45.8526, 54.3066) -> (45.8526, 54.3574) centre (45.8526, 54.332) ccw
  arc A102 (42.9204, 53.1509) -> (42.5958, 52.8264) centre (42.9204, 52.8263) ccw
  line L26 (43.7642, 52.8264) -> (43.7642, 52.5018)
  arc A103 (45.8526, 53.7083) -> (45.8526, 53.6575) centre (45.8526, 53.6829) ccw
  arc A104 (45.8526, 53.1763) -> (45.8526, 53.1255) centre (45.8526, 53.1509) ccw
  arc A105 (45.8526, 54.3574) -> (45.8526, 54.3066) centre (45.8526, 54.332) ccw
  arc A106 (45.2684, 53.7478) -> (45.2684, 54.2671) centre (45.2684, 54.0075) ccw
  arc A107 (43.7388, 52.8264) -> (43.7896, 52.8264) centre (43.7642, 52.8264) ccw
  arc A108 (45.3334, 53.1255) -> (45.3334, 53.1763) centre (45.3334, 53.1509) ccw
  arc A109 (44.9834, 52.5018) -> (45.0342, 52.5018) centre (45.0088, 52.5018) ccw
  arc A110 (45.2684, 54.2925) -> (45.2684, 54.2417) centre (45.2684, 54.2671) ccw
  arc A111 (45.2684, 53.7732) -> (45.2684, 53.7224) centre (45.2684, 53.7478) ccw
  arc A112 (42.9853, 53.6829) -> (43.2449, 53.9425) centre (42.9853, 53.9425) ccw
  arc A113 (42.9204, 53.6575) -> (42.9204, 53.7083) centre (42.9204, 53.6829) ccw
  arc A114 (42.9204, 54.3066) -> (42.9204, 54.3574) centre (42.9204, 54.332) ccw
  arc A115 (43.2449, 54.3066) -> (43.2449, 54.3574) centre (43.2449, 54.332) ccw
  arc A116 (43.2449, 54.3574) -> (43.2449, 54.3066) centre (43.2449, 54.332) ccw
  arc A117 (42.9204, 53.7083) -> (42.9204, 53.6575) centre (42.9204, 53.6829) ccw
  arc A118 (42.9853, 53.6575) -> (42.9853, 53.7083) centre (42.9853, 53.6829) ccw
  arc A119 (42.9204, 53.1763) -> (42.9204, 53.1255) centre (42.9204, 53.1509) ccw
  arc A120 (43.2703, 53.9425) -> (43.2195, 53.9425) centre (43.2449, 53.9425) ccw
  arc A121 (42.5704, 52.8264) -> (42.6212, 52.8264) centre (42.5958, 52.8264) ccw
  arc A122 (43.2703, 54.332) -> (43.2195, 54.332) centre (43.2449, 54.332) ccw
  line L27 (42.9853, 53.6829) -> (42.9204, 53.6829)
  line L28 (42.9204, 54.332) -> (43.2449, 54.332)
  arc A123 (43.7642, 53.8127) -> (43.2449, 54.332) centre (43.2449, 53.8127) ccw
  arc A124 (46.1772, 52.4764) -> (46.1772, 52.5272) centre (46.1772, 52.5018) ccw
  arc A125 (45.0342, 52.8264) -> (44.9834, 52.8264) centre (45.0088, 52.8264) ccw
  line L29 (42.9204, 53.1509) -> (43.4396, 53.1509)
  arc A126 (45.0088, 52.5272) -> (45.0088, 52.4764) centre (45.0088, 52.5018) ccw
  line L30 (45.0088, 52.5018) -> (45.0088, 52.8264)
  line L31 (45.3334, 53.1509) -> (45.8526, 53.1509)
  arc A127 (42.9204, 54.332) -> (42.9204, 53.6829) centre (42.9204, 54.0074) ccw
  arc A128 (43.7388, 52.5018) -> (43.7896, 52.5018) centre (43.7642, 52.5018) ccw
  arc A129 (45.3334, 53.1763) -> (45.3334, 53.1255) centre (45.3334, 53.1509) ccw
  arc A130 (46.1518, 52.8264) -> (46.2026, 52.8264) centre (46.1772, 52.8264) ccw
  arc A131 (43.7642, 52.8264) -> (43.4396, 53.1509) centre (43.4396, 52.8263) ccw
  line L32 (46.1772, 52.8264) -> (46.1772, 52.5018)
  arc A132 (45.3334, 53.1509) -> (45.0088, 52.8264) centre (45.3334, 52.8263) ccw
  arc A133 (45.8526, 53.6575) -> (45.8526, 53.7083) centre (45.8526, 53.6829) ccw
  arc A134 (43.7896, 52.8264) -> (43.7388, 52.8264) centre (43.7642, 52.8264) ccw
  arc A135 (46.1772, 52.8264) -> (45.8526, 53.1509) centre (45.8526, 52.8263) ccw
  arc A136 (42.9853, 53.7083) -> (42.9853, 53.6575) centre (42.9853, 53.6829) ccw
  arc A137 (45.2684, 54.2417) -> (45.2684, 54.2925) centre (45.2684, 54.2671) ccw
  arc A138 (45.2684, 53.7224) -> (45.2684, 53.7732) centre (45.2684, 53.7478) ccw
  arc A139 (42.5704, 52.5018) -> (42.6212, 52.5018) centre (42.5958, 52.5018) ccw
  arc A140 (43.4396, 53.1255) -> (43.4396, 53.1763) centre (43.4396, 53.1509) ccw
  arc A141 (43.2195, 53.9425) -> (43.2703, 53.9425) centre (43.2449, 53.9425) ccw
  line L33 (46.1772, 52.5018) -> (45.0088, 52.5018)
  arc A142 (45.8526, 53.1255) -> (45.8526, 53.1763) centre (45.8526, 53.1509) ccw
  arc A143 (42.5958, 52.5272) -> (42.5958, 52.4764) centre (42.5958, 52.5018) ccw
  arc A144 (42.9204, 53.1255) -> (42.9204, 53.1763) centre (42.9204, 53.1509) ccw
  arc A145 (42.9204, 54.3574) -> (42.9204, 54.3066) centre (42.9204, 54.332) ccw
  arc A146 (46.1518, 52.5018) -> (46.2026, 52.5018) centre (46.1772, 52.5018) ccw
  arc A147 (42.6212, 52.8264) -> (42.5704, 52.8264) centre (42.5958, 52.8264) ccw
  arc A148 (43.7388, 53.8127) -> (43.7896, 53.8127) centre (43.7642, 53.8127) ccw
  arc A149 (43.4396, 53.1763) -> (43.4396, 53.1255) centre (43.4396, 53.1509) ccw
  line L34 (43.2449, 54.332) -> (43.2449, 53.9425)
  arc A150 (44.9834, 52.8264) -> (45.0342, 52.8264) centre (45.0088, 52.8264) ccw
  arc A151 (43.7642, 52.4764) -> (43.7642, 52.5272) centre (43.7642, 52.5018) ccw
  arc A152 (45.8526, 53.6829) -> (45.8526, 54.332) centre (45.8526, 54.0074) ccw
  arc A153 (46.2026, 52.8264) -> (46.1518, 52.8264) centre (46.1772, 52.8264) ccw
  arc A154 (45.8526, 54.332) -> (45.8526, 53.6829) centre (45.8526, 54.0074) ccw
  arc A155 (45.2684, 54.2671) -> (45.2684, 53.7478) centre (45.2684, 54.0075) ccw
  arc A156 (51.0596, 54.3066) -> (51.0596, 54.3574) centre (51.0596, 54.332) ccw
  arc A157 (48.0004, 53.189) -> (48.0004, 53.2398) centre (48.0004, 53.2144) ccw
  line L35 (47.6758, 53.7464) -> (47.6758, 54.3955)
  arc A158 (50.5404, 53.1509) -> (50.2158, 52.8264) centre (50.5404, 52.8263) ccw
  arc A159 (47.6758, 52.5907) -> (47.6758, 52.5399) centre (47.6758, 52.5653) ccw
  arc A160 (50.2412, 54.2022) -> (50.1904, 54.2022) centre (50.2158, 54.2022) ccw
  arc A161 (51.0596, 53.6575) -> (51.0596, 53.7083) centre (51.0596, 53.6829) ccw
  arc A162 (47.6504, 53.7464) -> (47.7012, 53.7464) centre (47.6758, 53.7464) ccw
  line L36 (53.9242, 52.5018) -> (52.7558, 52.5018)
  arc A163 (47.7012, 52.8899) -> (47.6504, 52.8899) centre (47.6758, 52.8899) ccw
  arc A164 (47.6504, 52.5653) -> (47.7012, 52.5653) centre (47.6758, 52.5653) ccw
  arc A165 (48.5196, 53.189) -> (48.5196, 53.2398) centre (48.5196, 53.2144) ccw
  arc A166 (48.8188, 52.8899) -> (48.8696, 52.8899) centre (48.8442, 52.8899) ccw
  arc A167 (50.5404, 53.1763) -> (50.5404, 53.1255) centre (50.5404, 53.1509) ccw
  arc A168 (48.0004, 53.2144) -> (47.6758, 52.8899) centre (48.0004, 52.8898) ccw
  line L37 (51.3842, 52.8264) -> (51.3842, 52.5018)
  arc A169 (51.0596, 53.1763) -> (51.0596, 53.1255) centre (51.0596, 53.1509) ccw
  arc A170 (51.3588, 52.5018) -> (51.4096, 52.5018) centre (51.3842, 52.5018) ccw
  arc A171 (51.3842, 52.8264) -> (51.0596, 53.1509) centre (51.0596, 52.8263) ccw
  arc A172 (47.6826, 54.42) -> (47.669, 54.371) centre (47.6758, 54.3955) ccw
  arc A173 (50.1904, 52.8264) -> (50.2412, 52.8264) centre (50.2158, 52.8264) ccw
  line L38 (47.6758, 54.3955) -> (48.8442, 54.071)
  line L39 (50.5404, 53.1509) -> (51.0596, 53.1509)
  arc A174 (51.0596, 53.1255) -> (51.0596, 53.1763) centre (51.0596, 53.1509) ccw
  arc A175 (51.4096, 52.8264) -> (51.3588, 52.8264) centre (51.3842, 52.8264) ccw
  line L40 (48.8442, 52.8899) -> (48.8442, 52.5653)
  arc A176 (50.9947, 54.332) -> (50.7351, 54.0724) centre (50.9947, 54.0724) ccw
  arc A177 (50.7605, 54.0724) -> (50.7097, 54.0724) centre (50.7351, 54.0724) ccw
  arc A178 (47.7012, 54.3955) -> (47.6504, 54.3955) centre (47.6758, 54.3955) ccw
  arc A179 (50.9947, 54.3066) -> (50.9947, 54.3574) centre (50.9947, 54.332) ccw
  line L41 (50.9947, 54.332) -> (51.0596, 54.332)
  arc A180 (51.0596, 53.6829) -> (51.0596, 54.332) centre (51.0596, 54.0074) ccw
  arc A181 (47.6504, 52.8899) -> (47.7012, 52.8899) centre (47.6758, 52.8899) ccw
  line L42 (48.0004, 53.2144) -> (48.5196, 53.2144)
  arc A182 (48.5196, 53.2398) -> (48.5196, 53.189) centre (48.5196, 53.2144) ccw
  arc A183 (51.3842, 52.4764) -> (51.3842, 52.5272) centre (51.3842, 52.5018) ccw
  arc A184 (48.8374, 54.0465) -> (48.851, 54.0954) centre (48.8442, 54.0709) ccw
  arc A185 (51.3588, 52.8264) -> (51.4096, 52.8264) centre (51.3842, 52.8264) ccw
  arc A186 (48.8442, 52.8899) -> (48.5196, 53.2144) centre (48.5196, 52.8898) ccw
  arc A187 (51.0596, 54.3574) -> (51.0596, 54.3066) centre (51.0596, 54.332) ccw
  line L43 (50.2158, 52.5018) -> (50.2158, 52.8264)
  arc A188 (50.7351, 53.7083) -> (50.7351, 53.6575) centre (50.7351, 53.6829) ccw
  arc A189 (50.5404, 53.1255) -> (50.5404, 53.1763) centre (50.5404, 53.1509) ccw
  arc A190 (50.7351, 53.6575) -> (50.7351, 53.7083) centre (50.7351, 53.6829) ccw
  arc A191 (50.2158, 54.2022) -> (50.7351, 53.6829) centre (50.7351, 54.2022) ccw
  arc A192 (47.6758, 53.7718) -> (47.6758, 53.721) centre (47.6758, 53.7464) ccw
  arc A193 (50.2158, 52.5272) -> (50.2158, 52.4764) centre (50.2158, 52.5018) ccw
  arc A194 (50.1904, 52.5018) -> (50.2412, 52.5018) centre (50.2158, 52.5018) ccw
  arc A195 (50.7097, 54.0724) -> (50.7605, 54.0724) centre (50.7351, 54.0724) ccw
  arc A196 (50.9947, 54.3574) -> (50.9947, 54.3066) centre (50.9947, 54.332) ccw
  line L44 (47.6758, 52.5653) -> (47.6758, 52.8899)
  arc A197 (48.8696, 52.8899) -> (48.8188, 52.8899) centre (48.8442, 52.8899) ccw
  arc A198 (48.8442, 52.5399) -> (48.8442, 52.5907) centre (48.8442, 52.5653) ccw
  arc A199 (47.8056, 53.721) -> (47.8056, 53.7718) centre (47.8056, 53.7464) ccw
  line L45 (47.8056, 53.7464) -> (47.6758, 53.7464)
  arc A200 (48.0004, 53.2398) -> (48.0004, 53.189) centre (48.0004, 53.2144) ccw
  line L46 (51.3842, 52.5018) -> (50.2158, 52.5018)
  line L47 (48.8442, 52.5653) -> (47.6758, 52.5653)
  arc A201 (50.2412, 52.8264) -> (50.1904, 52.8264) centre (50.2158, 52.8264) ccw
  arc A202 (48.8188, 52.5653) -> (48.8696, 52.5653) centre (48.8442, 52.5653) ccw
  arc A203 (50.7097, 53.6829) -> (50.7605, 53.6829) centre (50.7351, 53.6829) ccw
  line L48 (50.7351, 53.6829) -> (50.7351, 54.0724)
  arc A204 (51.0596, 53.7083) -> (51.0596, 53.6575) centre (51.0596, 53.6829) ccw
  line L49 (51.0596, 53.6829) -> (50.7351, 53.6829)
  line L50 (56.4642, 52.5018) -> (55.2958, 52.5018)
  arc A205 (40.2263, 55.3536) -> (40.2098, 55.4017) centre (40.2181, 55.3776) ccw
  arc A206 (53.5996, 53.1255) -> (53.5996, 53.1763) centre (53.5996, 53.1509) ccw
  arc A207 (53.9496, 52.8264) -> (53.8988, 52.8264) centre (53.9242, 52.8264) ccw
  arc A208 (54.6885, 2.4638) -> (54.6885, 2.5146) centre (54.6885, 2.4892) ccw
  arc A209 (55.2704, 52.5018) -> (55.3212, 52.5018) centre (55.2958, 52.5018) ccw
  arc A210 (55.6204, 53.1255) -> (55.6204, 53.1763) centre (55.6204, 53.1509) ccw
  arc A211 (53.0804, 53.1509) -> (52.7558, 52.8264) centre (53.0804, 52.8263) ccw
  arc A212 (56.4388, 52.8264) -> (56.4896, 52.8264) centre (56.4642, 52.8264) ccw
  line L51 (52.7558, 52.5018) -> (52.7558, 52.8264)
  arc A213 (53.9242, 52.4764) -> (53.9242, 52.5272) centre (53.9242, 52.5018) ccw
  line L52 (26.0858, 30.353) -> (27.2542, 30.7425)
  arc A214 (54.4542, 1.5804) -> (54.4034, 1.5804) centre (54.4288, 1.5804) ccw
  line L53 (53.6646, 54.332) -> (53.5347, 54.332)
  arc A215 (26.8647, 29.8986) -> (26.8647, 29.9494) centre (26.8647, 29.924) ccw
  arc A216 (53.6646, 54.3066) -> (53.6646, 54.3574) centre (53.6646, 54.332) ccw
  arc A217 (53.5347, 54.3574) -> (53.5347, 54.3066) centre (53.5347, 54.332) ccw